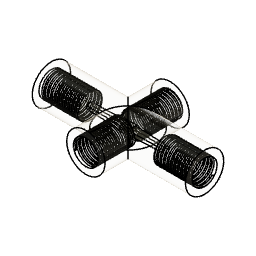
EC_sensor_one-part (Autodesk Fusion 360 design; units mm, degrees)
Autodesk Fusion 360 part; units mm, degrees
sketch "Skizze1" plane through (0, 0, 0) normal (0, 0, 1) x (1, 0, 0)
  line L0 (-20, 5) -> (-20, -5)
  line L1 (-20, -5) -> (-5, -5)
  line L2 (-5, -5) -> (-5, -11)
  line L3 (-5, -11) -> (5, -11)
  line L4 (5, -11) -> (5, -5)
  line L5 (5, -5) -> (20, -5)
  line L6 (-20, 5) -> (-5, 5)
  line L7 (-5, 5) -> (-5, 11)
  line L8 (-5, 11) -> (5, 11)
  line L9 (5, 11) -> (5, 5)
  line L10 (5, 5) -> (20, 5)
  line L11 (20, 5) -> (20, -5)
  line L12 (20, -5, 0) -> (20, -5, 10)
  line L13 (20, -5, 10) -> (20, 5, 10)
  line L14 (20, 5, 10) -> (20, 5, 0)
  line L15 (5, 5, 0) -> (5, 5, 10)
  line L16 (5, 5, 10) -> (20, 5, 10)
  line L17 (20, -5, 10) -> (5, -5, 10)
  line L18 (5, -5, 10) -> (5, -5, 0)
  line L19 (5, -11, 0) -> (5, -11, 10)
  line L20 (5, -11, 10) -> (-5, -11, 10)
  line L21 (12.4609, 50.9654) -> (12.4609, 50.3407)
  line L22 (5, -5, 10) -> (5, -11, 10)
  line L23 (-5, -11, 10) -> (-5, -11, 0)
  line L24 (-5, -5, 0) -> (-5, -5, 10)
  line L25 (-5, -5, 10) -> (-5, -11, 10)
  line L26 (-5, 5, 0) -> (-5, 5, 10)
  line L27 (-5, 5, 10) -> (-20, 5, 10)
  line L28 (-20, 5, 10) -> (-20, 5, 0)
  line L29 (-20, 5, 10) -> (-20, -5, 10)
  line L30 (-20, -5, 10) -> (-20, -5, 0)
  line L31 (-20, -5, 10) -> (-5, -5, 10)
  line L32 (5, 11, 0) -> (5, 11, 10)
  line L33 (5, 5, 10) -> (5, 11, 10)
  line L34 (-5, 11, 0) -> (-5, 11, 10)
  line L35 (5, 11, 10) -> (-5, 11, 10)
  line L36 (-5, 5, 10) -> (-5, 11, 10)
  constraint vertical L0
  constraint perpendicular L0 L1
  constraint perpendicular L1 L2
  constraint perpendicular L0 L3
  constraint perpendicular L3 L4
  constraint perpendicular L4 L5
  constraint perpendicular L0 L6
  constraint perpendicular L6 L7
  constraint perpendicular L7 L8
  constraint perpendicular L8 L9
  constraint perpendicular L9 L10
  constraint perpendicular L5 L11
  constraint perpendicular L8 L21
sketch "Skizze2" plane through (0, 0, 10) normal (0, 0, 1) x (1, 0, 0)
  line L0 (-1, 1, -5.5) -> (-1, -1, -5.5)
  line L1 (-1, -1, -5.5) -> (-1, -1, -4.5)
  line L2 (-1, -1, -4.5) -> (-1, 1, -4.5)
  line L3 (-1, 1, -4.5) -> (-1, 1, -5.5)
  line L4 (-1, 1, -5.5) -> (-1, -1, -4.5) construction
  line L5 (-1, -1, -5.5) -> (-1, 1, -4.5) construction
  line L6 (1, -1, -4.5) -> (1, 1, -4.5)
  line L7 (1, -1, -5.5) -> (1, -1, -4.5)
  line L8 (1, -1, -5.5) -> (1, 1, -4.5) construction
  line L9 (1, 1, -5.5) -> (1, -1, -5.5)
  line L10 (1, 1, -5.5) -> (1, -1, -4.5) construction
  line L11 (1, 1, -4.5) -> (1, 1, -5.5)
  line L12 (-1, -1, -4.5) -> (1, -1, -4.5)
  line L13 (-1, -1, -5.5) -> (1, -1, -5.5)
  line L14 (-1, 1, -4.5) -> (1, 1, -4.5)
  line L15 (1, 1, -5.5) -> (-1, 1, -5.5)
  circle A0 through (-10, 0.8, -5) (-10, -0.4, -4.3072) (-10, -0.4, -5.6928)
  circle A1 through (10, 0.8, -5) (10, -0.4, -4.3072) (10, -0.4, -5.6928)
  point P0 (-1, 0)
  point P1 (1, 0)
extrude "Extrusion1" add sketch "Skizze1" along normal blind 10
loft "Erhebung1" cut profiles "Skizze2", "Skizze2" section 1 contours L6 L7 L9 L11 in plane through (1, 0, 10) normal (1, 0, 0) section 2 contours A1 in plane through (10, 0, 10) normal (1, 0, 0)
loft "Erhebung2" cut profiles "Skizze2", "Skizze2" section 1 contours L0 L1 L2 L3 in plane through (-1, 0, 10) normal (1, 0, 0) section 2 contours A0 in plane through (-10, 0, 10) normal (1, 0, 0)
extrude "Extrusion2" cut sketch "Skizze2" against normal blind 2 contours L6 L7 L9 L11 in plane through (1, 0, 10) normal (1, 0, 0)
hole "Bohrung1" at (-20, 0, 5) direction (1, 0, 0) diameter 6.5 depth 10 tip angle 180
hole "Bohrung2" at (20, 0, 5) direction (-1, 0, 0) diameter 6.5 depth 10 tip angle 180
hole "Bohrung3" at (0, -11, 5) direction (0, 1, 0) diameter 6.5 depth 9.7 tip angle 180
hole "Bohrung4" at (0, 11, 5) direction (0, -1, 0) diameter 6.5 depth 9.7 tip angle 180
sketch "Skizze3" plane through (0, 0, 0) normal (0, 1, 0) x (1, 0, 0)
  line L0 (1, -4.5, 1.3) -> (-1, -4.5, 1.3)
  line L1 (-1, -4.5, 1.3) -> (-1, -5.5, 1.3)
  line L2 (-1, -5.5, 1.3) -> (1, -5.5, 1.3)
  line L3 (1, -5.5, 1.3) -> (1, -4.5, 1.3)
  line L4 (1, -4.5, 1.3) -> (-1, -5.5, 1.3) construction
  line L5 (-1, -4.5, 1.3) -> (1, -5.5, 1.3) construction
  line L6 (1, -5.5, -1.3) -> (-1, -5.5, -1.3)
  line L7 (-1, -5.5, -1.3) -> (-1, -4.5, -1.3)
  line L8 (-1, -4.5, -1.3) -> (1, -4.5, -1.3)
  line L9 (1, -4.5, -1.3) -> (1, -5.5, -1.3)
  line L10 (1, -5.5, -1.3) -> (-1, -4.5, -1.3) construction
  line L11 (-1, -5.5, -1.3) -> (1, -4.5, -1.3) construction
  point P0 (0, -5)
  point P1 (0, -5)
extrude "Extrusion5" cut sketch "Skizze3" along normal blind 0.3 contours L6 L7 L8 L9 in plane through (0, -1.3, 0) normal (0, 1, 0)
extrude "Extrusion6" cut sketch "Skizze3" against normal blind 0.3 contours L0 L1 L2 L3 in plane through (0, 1.3, 0) normal (0, 1, 0)
coil "Grundkörper Spirale1" add diameter 6.5 section triangle in size 0.4 inside turns 10.55556 pitch 0.9 right hand placed x (1, 0, 0) y (0, 0, 1) z (0, -1, 0) at (0, -1.3, 5)
coil "Grundkörper Spirale2" add diameter 6.5 section triangle in size 0.4 inside turns 10.88889 pitch 0.9 right hand placed x (0, 1, 0) y (0, 0, 1) z (1, 0, 0) at (10, 0, 5)
coil "Grundkörper Spirale3" add diameter 6.5 section triangle in size 0.4 inside turns 10.88889 pitch 0.9 right hand placed x (0, -1, 0) y (0, 0, 1) z (-1, 0, 0) at (-10, 0, 5)
coil "Grundkörper Spirale4" add diameter 6.5 section triangle in size 0.4 inside turns 10.55556 pitch 0.9 right hand placed x (-1, 0, 0) y (0, 0, 1) z (0, 1, 0) at (0, 1.3, 5)
delete_face "Fläche löschen1" 1 faces at (-3.0756, -11.0178, 3.9497)
delete_face "Fläche löschen2" 1 faces at (3.0756, 11.0178, 3.9497)
delete_face "Fläche löschen3" 1 faces at (-20.0178, -2.4474, 2.8616)
delete_face "Fläche löschen4" 1 faces at (20.0178, 2.4474, 2.8616)
fillet "Abrundung1" radius 5 16 edges at (-12.5, -5, 10) (-5, -8, 10) (5, -8, 10) (5, 8, 10) (-5, 8, 10) (-12.5, 5, 10) (12.5, 5, 10) (12.5, -5, 10) (5, -8, 0) (12.5, -5, 0) (-5, -8, 0) (-12.5, -5, 0) (-12.5, 5, 0) (-5, 8, 0) (12.5, 5, 0) (5, 8, 0)
sketch "Sketch11" plane through (0, 0, 0) normal (0, 0, 1) x (1, 0, 0)
